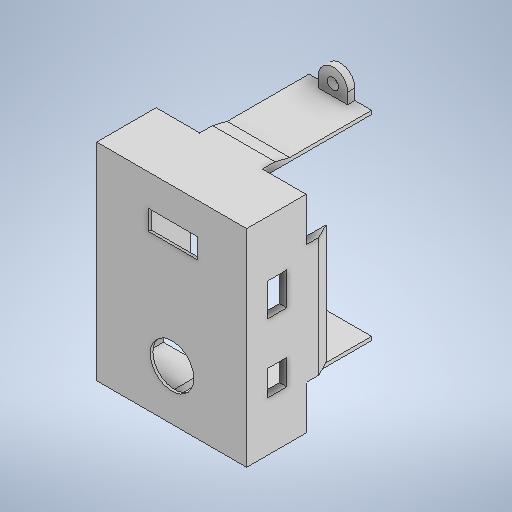
# Autodesk Inventor part: conn_enclosure
Saved by Autodesk Inventor 2025.1 (Build 291241000, 241)
## iProperties
Created: 2025-05-02
Part Number: conn_enclosure
Material: Generic
Document SubType Name: Modeling
Designer: santiago
Density: 1 g/cm^3
Appearance: Default
Author: santiago
Autodesk Inventor part; units mm, degrees
sketch "Sketch1" plane through (0, 0, 0) normal (0, 0, 1) x (1, 0, 0)
  line L0 (20.5, 16.5) -> (20.5, 28.5) projected
  line L1 (20.5, 28.5) -> (8.5, 28.5) projected
  line L2 (-20.7, -28.3) -> (-8.7, -28.3) projected
  line L3 (-20.7, -16.3) -> (-20.7, -28.3) projected
  line L4 (20.5, 28.5) -> (-20.7, 28.5)
  line L5 (-20.7, 28.5) -> (-20.7, -28.3)
  line L6 (-20.7, -28.3) -> (20.5, -28.3)
  line L7 (20.5, -28.3) -> (20.5, 28.5)
  point P0 (0, 0)
  constraints: 8 end point, 2 parallel, 1 horizontal, 1 perpendicular
extrude "Extrusion1" add sketch "Sketch1" along normal blind 4 and the other way blind 42.33
sketch "Sketch2" plane through (0, 0, -42.33) normal (0, 0, -1) x (-1, 0, 0)
  line L0 (18.8, 26.6) -> (-18.6, 26.6) projected
  line L1 (-18.5, 26.5) -> (-8.5, 26.5) projected
  line L2 (-18.5, 16.5) -> (-18.5, 26.5) projected
  line L3 (18.7, -16.3) -> (18.7, -26.3) projected
  line L4 (18.7, -26.3) -> (8.7, -26.3) projected
  line L5 (-18.5, 26.5) -> (18.7, 26.5)
  line L6 (18.7, 26.5) -> (18.7, -26.3)
  line L7 (18.7, -26.3) -> (-18.5, -26.3)
  line L8 (-18.5, -26.3) -> (-18.5, 26.5)
  point P0 (0, 0)
  constraints: 8 end point, 2 parallel, 1 horizontal, 1 perpendicular
extrude "Extrusion2" cut sketch "Sketch2" against normal blind 45.6
sketch "Sketch3" plane through (0, 0, -42.33) normal (0, 0, -1) x (-1, 0, 0)
  line L0 (8.7, 28.5) -> (20.7, 28.5)
  line L1 (20.7, 28.5) -> (20.7, -28.3)
  line L2 (20.7, -28.3) -> (8.7, -28.3)
  line L3 (8.7, -28.3) -> (8.7, 28.5)
  line L4 (-8.5, -28.3) -> (-20.5, -28.3)
  line L5 (-20.5, -28.3) -> (-20.5, 28.5)
  line L6 (-20.5, 28.5) -> (-8.5, 28.5)
  line L7 (-8.5, 28.5) -> (-8.5, -28.3)
  point P0 (0, 0)
  constraints: 16 end point, 4 parallel, 2 horizontal, 2 perpendicular, 4 other
ref_plane "Work Plane1" through (-20.7, 16.5, -12.33) normal (0, 0, 1) x (1, 0, 0)
extrude "Extrusion3" cut sketch "Sketch3" against normal up to surface (30 mm away)
sketch "Sketch4" plane through (0, 0, 4) normal (0, 0, 1) x (1, 0, 0)
  line L0 (-2.965, 15.255) -> (3.505, 15.255) projected
  line L1 (2.05, 18.905) -> (-2.965, 18.905) projected
  line L2 (-3.025, 18.845) -> (-3.025, 18.0225) projected
  line L3 (3.63, 17.715) -> (3.63, 18.845) projected
  line L4 (0.07, 16.645) -> (0.47, 16.645) projected
  line L5 (0.07, 17.515) -> (0.47, 17.515) projected
  line L6 (0.27, 16.645) -> (0.27, 17.515)
  line L7 (7.02, 19.83) -> (-6.48, 19.83)
  line L8 (-6.48, 19.83) -> (-6.48, 14.33)
  line L9 (-6.48, 14.33) -> (7.02, 14.33)
  line L10 (7.02, 14.33) -> (7.02, 19.83)
  line L11 (7.02, 19.83) -> (-6.48, 14.33) construction
  line L12 (-6.48, 19.83) -> (7.02, 14.33) construction
  point P0 (0, 0)
  point P1 (0.27, 17.08)
  dimension "d16" = 13.5
  dimension "d17" = 5.5
  constraints: 14 end point, 5 midpoint, 2 parallel, 1 horizontal, 1 perpendicular
  measures "d16" distance of L9.end L8.end
  measures "d17" distance of L8.end L7.end
extrude "Extrusion4" cut sketch "Sketch4" against normal through all
sketch "Sketch6" plane through (18.5, -26.3, 3.27) normal (-1, 0, 0) x (0, 0, 1)
  line L0 (-8.265, 35.2) -> (-8.265, 34.7) projected
  line L1 (-7.715, 14.39) -> (-8.265, 14.39) projected
  line L2 (-7.715, 15.89) -> (-8.265, 15.89) projected
  line L3 (-7.99, 14.39) -> (-7.99, 15.89)
  line L4 (-9.715, 14.89) -> (-9.715, 15.39) projected
  line L5 (-4.88, 52.7) -> (-4.88, -0.1) projected
  line L6 (-9.715, 36.4) -> (-9.715, 33.5) projected
  line L7 (-9.715, 15.14) -> (-4.88, 15.14)
  line L8 (-9.715, 34.95) -> (-4.88, 34.95)
  line L9 (-4.2975, 11.64) -> (-10.2975, 11.64)
  line L10 (-10.2975, 11.64) -> (-10.2975, 18.64)
  line L11 (-10.2975, 18.64) -> (-4.2975, 18.64)
  line L12 (-4.2975, 18.64) -> (-4.2975, 11.64)
  line L13 (-4.2975, 11.64) -> (-10.2975, 18.64) construction
  line L14 (-10.2975, 11.64) -> (-4.2975, 18.64) construction
  line L15 (-4.2975, 30.45) -> (-10.2975, 30.45)
  line L16 (-10.2975, 30.45) -> (-10.2975, 39.45)
  line L17 (-10.2975, 39.45) -> (-4.2975, 39.45)
  line L18 (-4.2975, 39.45) -> (-4.2975, 30.45)
  line L19 (-4.2975, 30.45) -> (-10.2975, 39.45) construction
  line L20 (-10.2975, 30.45) -> (-4.2975, 39.45) construction
  point P0 (-3.27, 26.3)
  point P1 (-7.2975, 15.14)
  point P2 (-7.2975, 34.95)
  point P3 (-4.88, 18.64)
  point P4 (-4.88, 11.64)
  point P5 (-4.88, 39.45)
  point P6 (-4.88, 30.45)
  dimension "d18" = 6
  dimension "d19" = 7
  dimension "d20" = 6
  dimension "d21" = 9
  constraints: 30 end point, 10 midpoint, 5 parallel, 3 perpendicular, 2 horizontal, 2 point on line
  measures "d18" distance of L10.end L11.end
  measures "d19" distance of L9.end L10.end
  measures "d20" distance of L16.end L17.end
  measures "d21" distance of L15.end L16.end
extrude "Extrusion5" cut sketch "Sketch6" against normal through all contours L5 L15 L16 L17 | L5 L9 L10 L11
sketch "Sketch7" plane through (-20.7, -28.3, 4) normal (-1, 0, 0) x (0, 0, 1)
  line L0 (-5.61, 41.45) -> (-5.61, 32.45) projected
  line L1 (-11.0275, 41.45) -> (-5.61, 41.45) projected
  line L2 (-5.61, 32.45) -> (-11.0275, 32.45) projected
  line L3 (-11.0275, 32.45) -> (-11.0275, 41.45) projected
  point P0 (-4, 28.3)
extrude "Extrusion6" cut sketch "Sketch7" against normal through all
sketch "Sketch8" plane through (-18.7, -26.3, 3.27) normal (0, 1, 0) x (1, 0, 0)
  line L0 (37.3, 4.88) -> (0.1, 4.88) projected
  line L1 (17.95, 9.715) -> (19.45, 9.715) projected
  line L2 (18.7, 9.715) -> (18.7, 4.88)
  line L3 (24.7, 2.7975) -> (12.7, 2.7975)
  line L4 (12.7, 2.7975) -> (12.7, 11.7975)
  line L5 (12.7, 11.7975) -> (24.7, 11.7975)
  line L6 (24.7, 11.7975) -> (24.7, 2.7975)
  line L7 (24.7, 2.7975) -> (12.7, 11.7975) construction
  line L8 (12.7, 2.7975) -> (24.7, 11.7975) construction
  point P0 (18.7, 3.27)
  point P1 (18.7, 7.2975)
  point P2 (24.7, 4.88)
  point P3 (12.7, 4.88)
  dimension "d26" = 12
  dimension "d27" = 9
  constraints: 14 end point, 5 midpoint, 2 parallel, 1 horizontal, 1 perpendicular
  measures "d26" distance of L4.end L5.end
  measures "d27" distance of L3.end L4.end
extrude "Extrusion7" cut sketch "Sketch8" against normal through all contours L0 L4 L5 L6
sketch "Sketch9" plane through (0, 0, -42.33) normal (0, 0, -1) x (-1, 0, 0)
  arc A0 (4.1, 30.5) -> (-3.9, 30.5) centre (0.1, 30.5) ccw projected
  line L0 (-3.9, 30.5) -> (-3.9, 27.5) projected
  line L1 (4.1, 27.5) -> (-3.9, 27.5) projected
  line L2 (4.1, 27.5) -> (4.1, 30.5) projected
  circle A1 centre (0.1, 30.5) radius 1.55 projected
  line L3 (-3.9, -27.3) -> (4.1, -27.3) projected
  line L4 (-3.9, -27.3) -> (-3.9, -30.3) projected
  arc A2 (-3.9, -30.3) -> (4.1, -30.3) centre (0.1, -30.3) ccw projected
  line L5 (4.1, -30.3) -> (4.1, -27.3) projected
  circle A3 centre (0.1, -30.3) radius 1.55 projected
  point P0 (0, 0)
extrude "Extrusion8" add sketch "Sketch9" against normal blind 2
thicken "Thicken2" operation cut thickness 1 both sides no extend neighbours no toward (0, 1, 0) faces at (1.2333, -28.3, -21.6633)
thicken "Thicken3" operation cut thickness 1 both sides no extend neighbours no toward (0, -1, 0) faces at (2.7667, 28.5, -1.4433)
ref_plane "Work Plane2" through (-18.7, 0.1, 3.27) normal (0, 1, 0) x (1, 0, 0)
sketch "Sketch10" plane through (-18.7, 0.1, 3.27) normal (0, 1, 0) x (1, 0, 0)
  line L0 (37.2, 17.6) -> (37.2, 23.1) projected
  line L1 (39.2, 19.1) -> (37.2, 23.1) projected
  line L2 (39.2, 19.1) -> (39.2, 15.6) projected
  line L3 (27.2, 15.6) -> (39.2, 15.6) projected
  line L4 (-2, 19.1) -> (0, 23.1) projected
  line L5 (0, 17.6) -> (0, 23.1) projected
  line L6 (-2, 15.6) -> (-2, 19.1) projected
  line L7 (-2, 15.6) -> (10, 15.6) projected
  line L8 (37.2, 17.6) -> (37.2, 15.6)
  line L9 (0, 17.6) -> (0, 15.6)
  point P0 (18.7, 3.27)
  constraints: 4 end point, 2 perpendicular, 2 point on line
extrude "Extrusion9" add sketch "Sketch10" along normal mid plane 32.77
sketch "Sketch12" plane through (8.5, 26.5, -12.33) normal (1, 0, 0) x (0, 0, -1)
  line L0 (3.5, 2) -> (0, 2)
  line L1 (3.5, 2) -> (7.5, 1)
  line L2 (30, 1) -> (0, 1) projected
  line L3 (0, -10) -> (0, 2)
  line L4 (3.5, -54.8) -> (7.5, -53.8)
  line L5 (0, -53.8) -> (30, -53.8) projected
  line L6 (3.5, -54.8) -> (0, -54.8)
  line L7 (0, -54.8) -> (0, -42.8)
  point P0 (-12.33, -26.5)
  constraints: 12 end point
ref_plane "Work Plane3" through (-8.7, 26.5, -42.35) normal (1, 0, 0) x (0, 1, 0)
extrude "Extrusion10" add sketch "Sketch12" against normal up to surface (17.2 mm away)
thicken "Thicken4" operation add thickness 1 both sides no extend neighbours no toward (0, 1, 0) faces at (2.7667, 27.5, -1.4433)
thicken "Thicken5" operation add thickness 1 both sides no extend neighbours no toward (0, -1, 0) faces at (-15.8, -27.3, -3.3133)
sketch "Sketch13" plane through (18.5, -26.3, 3.27) normal (-1, 0, 0) x (0, 0, 1)
  line L0 (-3.32, 0.0099) -> (-3.32, 52.8099) projected
  line L1 (-3.32, 47.5327) -> (-1.32, 47.5327)
  line L2 (-1.32, 47.5327) -> (-1.32, 2.5327)
  line L3 (-1.32, 2.5327) -> (-3.32, 2.5327)
  line L4 (-3.32, 2.5327) -> (-3.32, 47.5327)
  point P0 (-3.27, 26.3)
  dimension "d44" = 2
  dimension "d45" = 45
  constraints: 8 end point, 2 parallel, 1 horizontal, 1 perpendicular, 1 point on line
  measures "d44" distance of L2.end L3.end
  measures "d45" distance of L1.end L2.end
extrude "Extrusion11" add sketch "Sketch13" along normal blind 1
chamfer "Chamfer1" distance 1 angle 45 1 edges at (17.5, -1.2673, 1.95)
ref_plane "Work Plane4" through (-0.1, -28.3, -12.33) normal (-1, 0, 0) x (0, 0, 1)
mirror "Mirror1" about plane through (-0.1, -28.3, -12.33) normal (-1, 0, 0) of "Extrusion11", "Chamfer1"
sketch "Sketch14" plane through (0, 0, 4) normal (0, 0, 1) x (1, 0, 0)
  circle A0 centre (0, -14.4386) radius 6
  point P0 (0, 0)
  dimension "d51" = 12
  constraints: 1 centre point
  measures "d51" diameter of A0
extrude "Extrusion12" cut sketch "Sketch14" against normal through all
body "Solid1"
